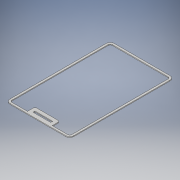
# Autodesk Inventor part: Rost_Basis
Saved by Autodesk Inventor 2018 (Build 220112000, 112)
## iProperties
Created: 2017-10-08
Part Number: Rost_Basis
Material: Generisch
Document SubType Name: Blech
Designer: Jan
Density: 1 g/cm^3
Sheet Metal Rule: Standard_mm
Appearance: Vorgabe
Author: Jan
Autodesk Inventor part; units mm, degrees
ref_plane "YZ Plane" through (0, 0, 0) normal (1, 0, 0) x (0, 1, 0)
ref_plane "XZ Plane" through (0, 0, 0) normal (0, 1, 0) x (-1, 0, 0)
ref_plane "XY Plane" through (0, 0, 0) normal (0, 0, 1) x (1, 0, 0)
sketch "Skizze1" plane through (0, 0, 0) normal (0, 0, 1) x (1, 0, 0)
  line L0 (-81, 132.5) -> (81, 132.5)
  line L1 (81, 132.5) -> (81, -132.5)
  line L2 (81, -132.5) -> (-81, -132.5)
  line L3 (-81, -132.5) -> (-81, 132.5)
  line L4 (-81, 132.5) -> (81, -132.5) construction
  line L5 (81, 132.5) -> (-81, -132.5) construction
  point P0 (0, 0)
  dimension "d0" = 162
  dimension "d1" = 265
  measures "d0" distance of L1.end L2.end
  measures "d1" distance of L0.end L1.end
extrude "Grobblech1" add sketch "Skizze1" along normal blind 2
fillet "Eckenrundung1" radius 10 4 edges at (-81, 132.5, 1) (81, 132.5, 1) (81, -132.5, 1) (-81, -132.5, 1)
sketch "Skizze2" plane through (0, 0, 2) normal (0, 0, 1) x (1, 0, 0)
  arc A0 (-81, -122.5) -> (-71, -132.5) centre (-71, -122.5) ccw projected
  line L0 (71, -132.5) -> (-71, -132.5) projected
  arc A1 (71, -132.5) -> (81, -122.5) centre (71, -122.5) ccw projected
  line L1 (81, 122.5) -> (81, -122.5) projected
  arc A2 (81, 122.5) -> (71, 132.5) centre (71, 122.5) ccw projected
  line L2 (-71, 132.5) -> (71, 132.5) projected
  arc A3 (-71, 132.5) -> (-81, 122.5) centre (-71, 122.5) ccw projected
  line L3 (-81, -122.5) -> (-81, 122.5) projected
  arc A4 (76, 122.5) -> (71, 127.5) centre (71, 122.5) ccw
  line L4 (76, 122.5) -> (76, -122.5)
  arc A5 (71, -127.5) -> (76, -122.5) centre (71, -122.5) ccw
  line L5 (71, -127.5) -> (-71, -127.5)
  arc A6 (-76, -122.5) -> (-71, -127.5) centre (-71, -122.5) ccw
  line L6 (-76, -122.5) -> (-76, 122.5)
  arc A7 (-71, 127.5) -> (-76, 122.5) centre (-71, 122.5) ccw
  line L7 (-71, 127.5) -> (71, 127.5)
  line L8 (-135.5785, 0) -> (231.9734, 0) projected
  line L9 (0, -191.312) -> (0, 205.8747) projected
  line L10 (-22.5, -117.5) -> (22.5, -117.5)
  line L11 (22.5, -117.5) -> (22.5, -122.5)
  line L12 (22.5, -122.5) -> (-22.5, -122.5)
  line L13 (-22.5, -122.5) -> (-22.5, -117.5)
  line L14 (30, -127.5) -> (30, -108.5)
  line L15 (30, -108.5) -> (-30, -108.5)
  line L16 (-30, -108.5) -> (-30, -127.5)
  line L17 (-53.5621, 127.5) -> (-20.4158, 127.5) construction
  point P0 (0, 0)
  dimension "d4" = 5
  dimension "d7" = 45
  dimension "d8" = 5
  dimension "d10" = 9
  dimension "d70" = 10
  dimension "d71" = 60
  constraints: 24 end point, 8 point on circle, 4 centre point, 3 parallel, 3 point on line, 2 horizontal, 2 perpendicular, 9 other
  measures "d4" distance between parallel lines of L2 L7
  measures "d7" distance of L11.end L12.end
  measures "d8" distance of L10.end L11.end
  measures "d10" distance between parallel lines of L15 L10
  measures "d70" distance between parallel lines of L0 L12
  measures "d71" distance of L14.end L15.end
extrude "Ausklinkung1" cut sketch "Skizze2" against normal blind 2 contours L12 L13 L10 L9 | L9 L10 L11 L12
sketch "Skizze5" plane through (0, 0, 2) normal (0, 0, 1) x (1, 0, 0)
  line L0 (-22.5, -122.5) -> (-22.5, -117.5) projected
  line L1 (-22.5, -117.5) -> (22.5, -117.5) projected
  line L2 (22.5, -117.5) -> (22.5, -122.5) projected
  line L3 (22.5, -122.5) -> (-22.5, -122.5) projected
  arc A0 (-81, -122.5) -> (-71, -132.5) centre (-71, -122.5) ccw projected
  line L4 (71, -132.5) -> (-71, -132.5) projected
  arc A1 (71, -132.5) -> (81, -122.5) centre (71, -122.5) ccw projected
  line L5 (81, 122.5) -> (81, -122.5) projected
  arc A2 (81, 122.5) -> (71, 132.5) centre (71, 122.5) ccw projected
  line L6 (-71, 132.5) -> (71, 132.5) projected
  arc A3 (-71, 132.5) -> (-81, 122.5) centre (-71, 122.5) ccw projected
  line L7 (-81, -122.5) -> (-81, 122.5) projected
  arc A4 (-71, 127.5) -> (-76, 122.5) centre (-71, 122.5) ccw
  line L8 (-71, 127.5) -> (71, 127.5)
  arc A5 (76, 122.5) -> (71, 127.5) centre (71, 122.5) ccw
  line L9 (76, 122.5) -> (76, -122.5)
  arc A6 (71, -127.5) -> (76, -122.5) centre (71, -122.5) ccw
  line L10 (71, -127.5) -> (-71, -127.5)
  arc A7 (-76, -122.5) -> (-71, -127.5) centre (-71, -122.5) ccw
  line L11 (-76, -122.5) -> (-76, 122.5)
  line L12 (26.5, -108.5) -> (-26.5, -108.5)
  line L13 (-31.5, -113.5) -> (-31.5, -132.5)
  line L14 (-31.5, -132.5) -> (31.5, -132.5)
  line L15 (31.5, -132.5) -> (31.5, -113.5)
  line L16 (-81, -122.5) -> (-81, 122.5) projected
  line L17 (31.5, -127.5) -> (-31.5, -127.5)
  line L18 (-31.5, -127.5) -> (-31.5, -113.5)
  line L19 (-26.5, -108.5) -> (26.5, -108.5)
  line L20 (31.5, -113.5) -> (31.5, -127.5)
  arc A8 (-26.5, -108.5) -> (-31.5, -113.5) centre (-26.5, -113.5) ccw
  arc A9 (31.5, -113.5) -> (26.5, -108.5) centre (26.5, -113.5) ccw
  line L21 (71, -132.5) -> (-71, -132.5) projected
  point P0 (0, 0)
  point P1 (31.5, -108.5)
  dimension "d37" = 5
  dimension "d38" = 9
  dimension "d41" = 5
  constraints: 24 end point, 12 point on circle, 6 centre point, 4 point on line, 4 tangent, 2 horizontal, 2 parallel, 1 collinear, 1 equal radius, 1 perpendicular, 7 other
  measures "d37" distance between parallel lines of L7 L11
  measures "d38" distance between parallel lines of L1 L12
  measures "d41" radius of A8
extrude "Ausklinkung2" cut sketch "Skizze5" against normal blind 2 contours L10 A7 L11 A4 L8 A5 L9 A6 L15 A9 L12 A8 L13
equation "\"d17\" = Stärke"
equation "\"d39\" = Stärke"
equation "\"d2\" = Stärke"
equation "\"Biegeradius\" = Stärke"
equation "\"BreiteBiegungsfreistellung\" = Stärke"
equation "\"TiefeBiegungsfreistellung\" = 0.5 * Stärke"
equation "\"GrößeEckenfreistellung\" = 4 * Stärke"
equation "\"MinimalRest\" = 2 * Stärke"
equation "\"Übergangsradius\" = Biegeradius"
equation "\"JacobiRadiusGröße\" = Biegeradius"
equation "\"Abstandsgröße\" = Stärke"
equation "\"Stärke\" = 2"
